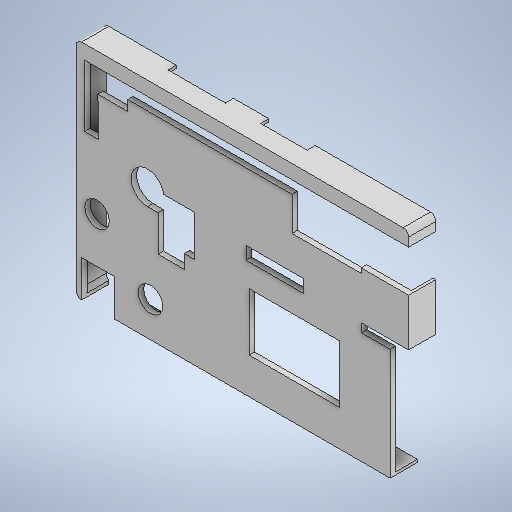
# Autodesk Inventor part: tampa_KiiRA
Saved by Autodesk Inventor 2026.3 (Build 303398000, 398)
## iProperties
Created: 2026-05-20
Part Number: tampa_KiiRA
Material: Genérico
Document SubType Name: Modeling
Designer: franciscowilke
Density: 1 g/cm^3
Appearance: Padrão
Author: franciscowilke
Autodesk Inventor part; units mm, degrees
ref_plane "YZ Plane" through (0, 0, 0) normal (1, 0, 0) x (0, 1, 0)
ref_plane "XZ Plane" through (0, 0, 0) normal (0, 1, 0) x (-1, 0, 0)
ref_plane "XY Plane" through (0, 0, 0) normal (0, 0, 1) x (1, 0, 0)
sketch "Esboço2" plane through (0, 0, 0) normal (0, 0, 1) x (1, 0, 0)
  line L0 (60.2596, 45.3747) -> (-61.7404, 45.3747)
  line L1 (-61.7404, 45.3747) -> (-61.7404, -36.6253)
  line L2 (-61.7404, -36.6253) -> (60.2596, -36.6253)
  line L3 (60.2596, -36.6253) -> (60.2596, 45.3747)
  line L4 (60.2596, 45.3747) -> (-61.7404, -36.6253) construction
  line L5 (-61.7404, 45.3747) -> (60.2596, -36.6253) construction
  point P0 (0, 0)
  dimension "d9" = 122
  dimension "d10" = 82
  constraints: 12 end point, 2 parallel, 1 horizontal, 1 perpendicular
  measures "d9" distance of L2.end L1.end
  measures "d10" distance of L1.end L0.end
extrude "Extrusão6" add sketch "Esboço2" against normal blind 10
sketch "Esboço11" plane through (0, 0, -10) normal (0, 0, -1) x (-1, 0, 0)
  line L0 (61.7404, -36.6253) -> (61.7404, 45.3747) construction
  line L1 (61.7404, 45.3747) -> (-60.2596, 45.3747) construction
  line L2 (-60.2596, 45.3747) -> (-60.2596, -36.6253) construction
  line L3 (-60.2596, -36.6253) -> (61.7404, -36.6253) construction
  line L4 (-60.2596, 45.3747) -> (61.7404, 45.3747)
  line L5 (61.7404, 45.3747) -> (61.7404, -36.6253)
  line L6 (61.7404, -36.6253) -> (-60.2596, -36.6253)
  line L7 (-60.2596, -36.6253) -> (-60.2596, 45.3747)
  line L8 (-59.2596, 44.3747) -> (60.7404, 44.3747)
  line L9 (60.7404, 44.3747) -> (60.7404, -35.6253)
  line L10 (60.7404, -35.6253) -> (-59.2596, -35.6253)
  line L11 (-59.2596, -35.6253) -> (-59.2596, 44.3747)
  point P0 (0, 0)
  dimension "d193" = 1
  constraints: 16 end point, 2 parallel, 1 horizontal, 1 perpendicular, 3 other
  measures "d193" distance between parallel lines of L1 L8
extrude "Extrusão8" cut sketch "Esboço11" against normal blind 8 contours L8 L9 L10 L11
sketch "Esboço4" plane through (0, 0, 0) normal (0, 0, 1) x (1, 0, 0)
  line L0 (17.4884, 35.5958) -> (-42.7686, 35.5958)
  line L1 (-58.5771, 17.7849) -> (-58.5771, -38.6492)
  line L2 (-58.5771, -38.6492) -> (53.4957, -38.6492)
  line L3 (-42.7686, 35.5958) -> (-42.7553, 31.7928)
  line L4 (-42.7553, 31.7928) -> (-53.7553, 31.7928)
  line L5 (-53.5771, 17.5439) -> (-53.7553, 31.7928)
  line L6 (34.9957, -23.3992) -> (1.7457, -23.3992)
  line L7 (1.7457, -23.3992) -> (1.7457, -2.2492)
  line L8 (1.7457, -2.2492) -> (34.9957, -2.2492)
  line L9 (34.9957, -2.2492) -> (34.9957, -23.3992)
  line L10 (53.4957, -38.6492) -> (53.4957, 4.3508)
  line L11 (53.4957, 4.3508) -> (43.0999, 4.3508)
  line L12 (43.0999, 4.3508) -> (43.0999, 7.5008)
  line L13 (21.6723, 6.2251) -> (0.6723, 6.2251)
  line L14 (0.6723, 6.2251) -> (0.6723, 10.9251)
  line L15 (0.6723, 10.9251) -> (21.6723, 10.9251)
  line L16 (21.6723, 10.9251) -> (21.6723, 6.2251)
  line L17 (-18.3453, -3.0069) -> (-22.0953, -3.0069)
  line L18 (-22.0953, -3.0069) -> (-22.0953, -8.0069)
  line L19 (-22.0953, -8.0069) -> (-31.6953, -8.0069)
  line L20 (-31.6953, -8.0069) -> (-31.6953, 5.1431)
  arc A0 (-29.6237, 11.9931) -> (-35.5632, 5.1431) centre (-35.5632, 11.1431) ccw
  line L21 (17.4884, 23.1519) -> (42.8384, 23.1519)
  line L22 (42.8384, 23.1519) -> (42.8384, 24.9019)
  circle A1 centre (-54.0634, -6.5069) radius 4.5
  circle A2 centre (-34.4514, -23.7569) radius 4.5
  line L23 (-34.4514, -23.7569) -> (-34.4514, -38.7569)
  line L24 (-34.4514, -23.7569) -> (-58.8894, -23.7569)
  line L25 (-54.0634, -6.5069) -> (-54.0634, -38.7569)
  line L26 (-54.0634, -6.5069) -> (-58.8894, -6.5069)
  line L27 (-35.5632, 11.1431) -> (-35.5632, -38.1569)
  line L28 (-35.5632, 11.1431) -> (-58.8892, 11.1431)
  line L29 (-18.3453, -3.0069) -> (-18.3453, 11.9931)
  line L30 (-18.3453, 11.9931) -> (-29.6237, 11.9931)
  line L31 (-35.5632, 5.1431) -> (-31.6953, 5.1431)
  line L32 (-58.5771, -38.6492) -> (58.6039, -38.6492)
  line L33 (-58.5771, 37.6428) -> (-58.5771, -38.6492)
  line L34 (17.4884, 23.1519) -> (17.4884, 35.5958)
  line L35 (42.8384, 24.9019) -> (61.4724, 24.9019)
  line L36 (43.0999, 7.5008) -> (61.4229, 7.5008)
  line L37 (-53.5771, 17.5439) -> (-58.5771, 17.5428)
  line L38 (58.6039, -38.6492) -> (58.6039, -28.6492)
  line L39 (-61.7404, -36.6253) -> (-61.7404, 45.3747) construction
  line L40 (-58.5771, -38.6492) -> (-58.5771, 40.1798)
  line L41 (-58.5771, 40.1798) -> (61.4229, 40.1798)
  line L42 (61.4229, 40.1798) -> (61.4229, -38.6492)
  line L43 (61.4229, -38.6492) -> (-58.5771, -38.6492)
  point P0 (0, 0)
  point P1 (53.4957, -38.6492)
  point P2 (53.4957, -38.6492)
  point P3 (61.4229, 24.9019)
  dimension "d101" = 33.25
  dimension "d102" = 21.15
  dimension "d109" = 15.25
  dimension "d132" = 43
  dimension "d139" = 3.15
  dimension "d146" = 21
  dimension "d147" = 4.7
  dimension "d152" = 3.75
  dimension "d153" = 5
  dimension "d154" = 9.6
  dimension "d172" = 9
  dimension "d173" = 9
  dimension "d176" = 3.803
  dimension "d180" = 60.257
  dimension "d184" = 6
  dimension "d199" = 32.25
  dimension "d200" = 4.826
  dimension "d201" = 23.326
  dimension "d205" = 15
  dimension "d206" = 13.15
  dimension "d214" = 12.4439
  dimension "d215" = 25.35
  dimension "d219" = 11
  dimension "d220" = 18.5
  dimension "d221" = 10
  dimension "d222" = 78.829
  dimension "d223" = 120
  dimension "d224" = 15
  dimension "d225" = 1.75
  dimension "d226" = 14.25
  dimension "d227" = 5
  constraints: 86 end point, 6 horizontal, 6 perpendicular, 4 parallel, 3 centre point, 3 point on line, 3 vertical, 2 point on circle, 1 collinear, 1 tangent
  measures "d101" distance of L7.end L8.end
  measures "d102" distance of L6.end L7.end
  measures "d109" distance between parallel lines of L2 L6
  measures "d132" distance of L2.end L10.end
  measures "d139" distance of L11.end L12.end
  measures "d146" distance of L14.end L15.end
  measures "d147" distance of L13.end L14.end
  measures "d152" distance of L17.start L17.end
  measures "d153" distance of L17.end L18.end
  measures "d154" distance of L18.end L19.end
  measures "d172" diameter of A1
  measures "d173" diameter of A2
  measures "d176" distance of L0.end L3.end
  measures "d180" distance of L0.start L0.end
  measures "d184" radius of A0
  measures "d199" distance of L25.start L25.end
  measures "d200" distance of L25.start L26.end
  measures "d201" distance of L27.start L28.end
  measures "d205" distance of L17.start L29.end
  measures "d206" distance of L19.end L20.end
  measures "d214" distance of L21.start L0.start
  measures "d215" distance of L21.start L21.end
  measures "d219" distance of L3.end L4.end
  measures "d220" distance between parallel lines of L10 L9
  measures "d221" distance of L32.end L38.end
  measures "d222" distance of L1.end L40.end
  measures "d223" distance of L40.end L41.end
  measures "d224" distance of L23.start L23.end
  measures "d225" distance of L21.end L22.end
  measures "d226" distance of L5.start L4.end
  measures "d227" distance of L5.start L37.end
fillet "Arredondamento3" radius 2 8 edges at (-60.7404, 44.3747, -6) (60.2596, -36.6253, -5) (-61.7404, -36.6253, -5) (-60.7404, -35.6253, -6) (-61.7404, 45.3747, -5) (60.2596, 45.3747, -5) (59.2596, 44.3747, -6) (59.2596, -35.6253, -6)
extrude "Extrusão10" cut sketch "Esboço4" against normal blind 20 contours L0 L3 L4 L5 L37 L1 L33 L40 L41 L42 L35 L22 L21 L34 | L42 L43 L32 L10 L11 L12 L36 | L28 L27 A0 | A0 L30 L29 L17 L18 L19 L20 L31 L27 L28 | L26 L25 A1 | A1 L25 L26 | L27 L24 A2 | A2 L23 L24 L27 | L24 L27 A2 | L24 L23 A2 L27 | L6 L7 L8 L9 | L13 L14 L15 L16
sketch "Esboço12" plane through (-59.7404, -36.6253, -10) normal (0, -1, 0) x (1, 0, 0)
  line L0 (113.2361, 0) -> (0, 0) construction
  line L1 (0, 10) -> (12, 10)
  line L2 (12, 10) -> (12, 0)
  line L3 (12, 0) -> (0, 0)
  line L4 (0, 0) -> (0, 10)
  point P0 (59.7404, 10)
  dimension "d230" = 12
  constraints: 8 end point, 2 parallel, 1 horizontal, 1 perpendicular, 1 point on line
  measures "d230" distance of L2.end L3.end
extrude "Extrusão11" cut sketch "Esboço12" against normal blind 13.5
sketch "Esboço13" plane through (-59.7404, 45.3747, 0) normal (0, 1, 0) x (1, 0, 0)
  line L0 (0, 10) -> (118, 10) construction
  line L1 (45.7717, 10) -> (24.7717, 10)
  line L2 (24.7717, 10) -> (24.7717, 7)
  line L3 (24.7717, 7) -> (45.7717, 7)
  line L4 (45.7717, 7) -> (45.7717, 10)
  line L5 (12, 10) -> (113.2361, 10) construction
  line L6 (58.7717, 10) -> (75.7717, 10)
  line L7 (75.7717, 10) -> (75.7717, 7)
  line L8 (75.7717, 7) -> (58.7717, 7)
  line L9 (58.7717, 7) -> (58.7717, 10)
  point P0 (59.7404, 0)
  point P1 (71.7717, 10)
  dimension "d233" = 21
  dimension "d235" = 3
  dimension "d241" = 17
  dimension "d243" = 3
  dimension "d244" = 13
  constraints: 16 end point, 4 parallel, 2 horizontal, 2 perpendicular, 2 point on line
  measures "d233" distance of L3.end L2.end
  measures "d235" distance of L3.end L1.start
  measures "d241" distance of L7.end L8.end
  measures "d243" distance of L8.end L6.start
  measures "d244" distance of L1.start L6.start
extrude "Extrusão12" cut sketch "Esboço13" against normal blind 18
